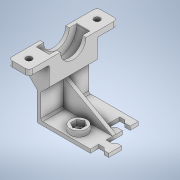
# Autodesk Inventor part: ДержательПодшипника_БН
Saved by Autodesk Inventor 2021 (Build 250183000, 183)
## iProperties
Created: 2023-02-11
Part Number: ДержательПодшипника_БН
Material: Типовые
Document SubType Name: Modeling
Designer: 1
Density: 1 g/cm^3
Appearance: По умолчанию
Author: 1
Autodesk Inventor part; units mm, degrees
ref_plane "YZ Plane" through (0, 0, 0) normal (1, 0, 0) x (0, 1, 0)
ref_plane "XZ Plane" through (0, 0, 0) normal (0, 1, 0) x (-1, 0, 0)
ref_plane "XY Plane" through (0, 0, 0) normal (0, 0, 1) x (1, 0, 0)
sketch "Эскиз1" plane through (0, 0, 0) normal (0, 0, 1) x (1, 0, 0)
  line L0 (0, 0) -> (-2, 0)
  line L1 (-2, 0) -> (-2, 20)
  line L2 (-2, 20) -> (0, 20)
  line L3 (0, 20) -> (0, 0)
  line L4 (-2, 0) -> (27, 0)
  line L5 (27, 0) -> (27, 2)
  line L6 (27, 2) -> (-2, 2)
  line L7 (-2, 2) -> (-2, 0)
  point P0 (0, 2)
  dimension "d4" = 2
  dimension "d5" = 20
  dimension "d6" = 2
  dimension "d7" = 27
  constraints: 16 end point, 4 parallel, 2 horizontal, 2 perpendicular
  measures "d4" distance of L1.end L2.end
  measures "d5" distance of L0.end L1.end
  measures "d6" distance of L5.end L4.end
  measures "d7" distance between parallel lines of L5 L3
extrude "Выдавливание1" add sketch "Эскиз1" along normal mid plane 26.1
sketch "Эскиз2" plane through (-2, 20, 13.05) normal (0, 1, 0) x (1, 0, 0)
  line L0 (4.55, 2) -> (-2.55, 2) construction
  line L1 (-2.55, 2) -> (-2.55, 24.1) construction
  line L2 (-2.55, 24.1) -> (4.55, 24.1) construction
  line L3 (4.55, 24.1) -> (4.55, 2) construction
  line L4 (4.55, 2) -> (-2.55, 24.1) construction
  line L5 (-2.55, 2) -> (4.55, 24.1) construction
  line L6 (2, 26.1) -> (2, 0) construction
  line L7 (0, 0) -> (0, 26.1) construction
  line L8 (2, 0) -> (0, 0) construction
  line L9 (2, 26.1) -> (2, 0) construction
  line L10 (0, 26.1) -> (2, 26.1) construction
  line L11 (6.55, 26.1) -> (-4.55, 26.1)
  line L12 (-4.55, 26.1) -> (-4.55, 0)
  line L13 (-4.55, 0) -> (6.55, 0)
  line L14 (6.55, 0) -> (6.55, 26.1)
  line L15 (6.55, 26.1) -> (-4.55, 0) construction
  line L16 (-4.55, 26.1) -> (6.55, 0) construction
  point P0 (2, 13.05)
  point P1 (1, 13.05)
  point P2 (1, 13.05)
  point P3 (2, 13.05)
  point P4 (1, 13.05)
  point P5 (1, 26.1)
  dimension "d10" = 7.1
  dimension "d11" = 22.1
  dimension "d12" = 2
  dimension "d13" = 2
  constraints: 24 end point, 8 midpoint, 4 parallel, 2 horizontal, 2 perpendicular, 1 horizontal alignment, 1 vertical alignment
  measures "d10" distance of L0.start L0.end
  measures "d11" distance of L0.end L1.end
  measures "d12" distance between parallel lines of L11 L2
  measures "d13" distance between parallel lines of L3 L14
extrude "Выдавливание2" add sketch "Эскиз2" along normal blind 13.5
shell "Оболочка1" thickness 2 removed faces 1 at (0.85, 33.5, -4.35)
fillet "Сопряжение1" radius 11 6 edges at (1.275, 22, -11.05) (-1, 22, -11.05) (-3.275, 22, -11.05) (-3.275, 22, 11.05) (-1, 22, 11.05) (1.275, 22, 11.05)
sketch "Эскиз3" plane through (-6.55, 20, -13.05) normal (-1, 0, 0) x (0, 0, 1)
  line L0 (26.1, 13.5) -> (0, 13.5) projected
  circle A0 centre (13.05, 13.5) radius 7
  point P0 (13.05, -20)
  point P1 (6.05, 13.5)
  point P2 (20.05, 13.5)
  dimension "d18" = 14
  constraints: 1 centre point, 1 midpoint
  measures "d18" diameter of A0
extrude "Выдавливание3" cut sketch "Эскиз3" against normal through all contours A0 L0 picked at (11.6567, 11.0213)
sketch "Эскиз4" plane through (0, 2, 13.05) normal (0, 1, 0) x (1, 0, 0)
  line L0 (27, 26.1) -> (27, 0) projected
  line L1 (27, 17.575) -> (24, 17.575)
  line L2 (24, 17.575) -> (22.5, 16.075)
  line L3 (22.5, 16.075) -> (20, 16.075)
  line L4 (27, 19.575) -> (10.0579, 19.575)
  line L5 (20, 16.075) -> (20, 19.575)
  line L6 (27, 21.575) -> (24, 21.575)
  line L7 (24, 21.575) -> (22.5, 23.075)
  line L8 (22.5, 23.075) -> (20, 23.075)
  line L9 (20, 23.075) -> (20, 19.575)
  line L10 (27, 13.05) -> (4.55, 13.05)
  line L11 (0, 26.1) -> (27, 26.1) projected
  line L12 (9.0322, 13.05) -> (9.0322, 26.1) construction
  line L13 (4.55, 20.05) -> (4.55, 6.05) projected
  line L14 (27, 8.525) -> (24, 8.525) construction
  line L15 (24, 8.525) -> (22.5, 10.025) construction
  line L16 (22.5, 10.025) -> (20, 10.025) construction
  line L17 (27, 6.525) -> (10.0579, 6.525)
  line L18 (20, 10.025) -> (20, 6.525) construction
  line L19 (27, 4.525) -> (24, 4.525) construction
  line L20 (24, 4.525) -> (22.5, 3.025) construction
  line L21 (22.5, 3.025) -> (20, 3.025) construction
  line L22 (20, 3.025) -> (20, 6.525) construction
  line L23 (31.5, 10.025) -> (34, 10.025)
  line L24 (30, 8.525) -> (31.5, 10.025)
  line L25 (27, 8.525) -> (30, 8.525)
  line L26 (34, 10.025) -> (34, 6.525)
  line L27 (27, 6.525) -> (43.9421, 6.525)
  line L28 (27, 4.525) -> (30, 4.525)
  line L29 (34, 3.025) -> (34, 6.525)
  line L30 (31.5, 3.025) -> (34, 3.025)
  line L31 (30, 4.525) -> (31.5, 3.025)
  line L32 (27, 4.525) -> (27, 8.525)
  line L33 (27, 17.575) -> (27, 21.575)
  point P0 (0, 13.05)
  point P1 (9.0322, 19.575)
  dimension "d21" = 3
  dimension "d22" = 7
  dimension "d23" = 2.5
  dimension "d24" = 4
  dimension "d25" = 7
  constraints: 62 end point, 23 symmetric about line, 7 point on line, 3 midpoint, 2 collinear, 2 horizontal, 2 perpendicular, 1 horizontal alignment, 1 parallel
  measures "d21" distance of L1.start L1.end
  measures "d22" distance between parallel lines of L8 L3
  measures "d23" distance of L2.end L3.end
  measures "d24" distance between parallel lines of L6 L1
  measures "d25" distance between parallel lines of L0 L9
extrude "Выдавливание4" add sketch "Эскиз4" against normal up to surface (2 mm away) contours L25 L24 L23 L26 L27 L0 | L27 L29 L30 L31 L28 L0
extrude "Выдавливание5" cut sketch "Эскиз4" against normal through all contours L0 L4 L9 L8 L7 L6 | L0 L1 L2 L3 L5 L4
sketch "Эскиз5" plane through (0, 0, 0) normal (0, 0, 1) x (1, 0, 0)
  line L0 (0, 17) -> (27, 2)
  point P0 (0, 0)
  point P1 (0, 20)
  dimension "d65" = 15
  constraints: 2 end point, 1 coincident, 1 vertical alignment
  measures "d65" vertical distance of L0.start L0.end
extrude "Ребро жесткости1" add sketch "Эскиз5" along normal mid plane 2 rib yes fills toward (13.4757, 9.4563) open curves L0
sketch "Эскиз6" plane through (-2, 33.5, 13.05) normal (0, 1, 0) x (1, 0, 0)
  line L0 (-4.55, 6.05) -> (-4.55, 20.05) projected
  line L1 (-4.55, 13.05) -> (30.5644, 13.05)
  line L2 (-4.55, 6.05) -> (-4.55, 0) projected
  line L3 (-4.55, 0) -> (6.55, 0)
  line L4 (6.55, 0) -> (6.55, -11.1)
  line L5 (6.55, -11.1) -> (-4.55, -11.1)
  line L6 (-4.55, -11.1) -> (-4.55, 0)
  circle A0 centre (1, -5.55) radius 1.6
  line L7 (-4.55, 26.1) -> (6.55, 26.1)
  line L8 (6.55, 26.1) -> (6.55, 37.2)
  line L9 (6.55, 37.2) -> (-4.55, 37.2)
  line L10 (-4.55, 37.2) -> (-4.55, 26.1)
  circle A1 centre (1, 31.65) radius 1.6
  point P0 (2, 13.05)
  point P1 (1, -11.1)
  point P2 (6.55, -5.55)
  point P3 (1, 37.2)
  point P4 (6.55, 31.65)
  dimension "d36" = 3.2
  constraints: 18 end point, 8 symmetric about line, 3 midpoint, 2 centre point, 2 coincident, 2 horizontal, 2 parallel, 2 perpendicular, 1 horizontal alignment, 1 vertical alignment, 1 other
  measures "d36" diameter of A0
extrude "Выдавливание6" add sketch "Эскиз6" against normal blind 3
fillet "Сопряжение2" radius 1 4 edges at (-1, 30.5, 13.05) (-1, 30.5, -13.05) (0, 2, -7.025) (0, 2, 7.025)
fillet "Сопряжение3" radius 0.5 1 edges at (-2, 0, 0)
chamfer "Фаска1" distance 4.55 angle 45 2 edges at (0, 20, 0) (-2, 20, 0)
sketch "Эскиз7" plane through (24, 2, -4.525) normal (0, 1, 0) x (1, 0, 0)
  line L0 (-4, -1.5) -> (-4, 5.5) projected
  line L1 (-1.5, -1.5) -> (-4, -1.5) projected
  line L2 (0, 0) -> (-1.5, -1.5) projected
  line L3 (3, 0) -> (0, 0) projected
  line L4 (0, 4) -> (3, 4) projected
  line L5 (-1.5, 5.5) -> (0, 4) projected
  line L6 (-4, 5.5) -> (-1.5, 5.5) projected
  line L7 (3, 0) -> (3, -3.525) projected
  line L8 (3, -0.1) -> (0.0414, -0.1)
  line L9 (0.0414, -0.1) -> (-1.4586, -1.6)
  line L10 (-1.4586, -1.6) -> (-4.1, -1.6)
  line L11 (-4.1, -1.6) -> (-4.1, 5.6)
  line L12 (-4.1, 5.6) -> (-1.4586, 5.6)
  line L13 (-1.4586, 5.6) -> (0.0414, 4.1)
  line L14 (0.0414, 4.1) -> (3, 4.1)
  line L15 (3, 8.525) -> (3, 4) projected
  point P0 (-24, -4.525)
  dimension "d44" = 0.1
  dimension "d45" = 0.1
  dimension "d46" = 0.1
  dimension "d47" = 0.1
  dimension "d48" = 0.1
  dimension "d49" = 0.1
  dimension "d50" = 0.1
  constraints: 14 end point, 4 parallel, 3 perpendicular, 2 point on line, 1 horizontal
  measures "d44" distance between parallel lines of L3 L8
  measures "d45" distance between parallel lines of L2 L9
  measures "d46" distance between parallel lines of L1 L10
  measures "d47" distance between parallel lines of L11 L0
  measures "d48" distance between parallel lines of L12 L6
  measures "d49" distance between parallel lines of L13 L5
  measures "d50" distance between parallel lines of L4 L14
extrude "Выдавливание7" cut sketch "Эскиз7" against normal through all
sketch "Эскиз8" plane through (1, 2, -13.05) normal (0, 1, 0) x (1, 0, 0)
  line L0 (26, -12.05) -> (26, -14.05) projected
  circle A0 centre (14, -20.55) radius 4.5
  line L1 (26, -21.575) -> (26, -26.1) projected
  line L2 (-1, -14.05) -> (-1, -26.1) projected
  line L3 (11.15, -18.9046) -> (14, -17.2591)
  line L4 (14, -17.2591) -> (16.85, -18.9046)
  line L5 (16.85, -18.9046) -> (16.85, -22.1954)
  line L6 (16.85, -22.1954) -> (14, -23.8409)
  line L7 (14, -23.8409) -> (11.15, -22.1954)
  line L8 (11.15, -22.1954) -> (11.15, -18.9046)
  line L9 (-7.55, 0) -> (-7.55, -26.1) projected
  point P0 (-1, -13.05)
  point P1 (-7.55, -13.05)
  dimension "d53" = 9
  dimension "d55" = 15
  dimension "d57" = 5.7
  dimension "d58" = 7.5
  constraints: 12 end point, 1 centre point, 1 coincident, 1 midpoint, 1 vertical, 13 other
  measures "d53" diameter of A0
  measures "d55" distance from line of L2 A0.centre
  measures "d57" distance between parallel lines of L8 L5
  measures "d58" vertical distance of A0.centre point (-7.55, -13.05)
extrude "Выдавливание8" add sketch "Эскиз8" along normal blind 3
sketch "Эскиз9" plane through (12.15, 2, 9.1454) normal (0, 1, 0) x (1, 0, 0)
  circle A0 centre (2.85, 1.6454) radius 1.6
  circle A1 centre (2.85, 1.6454) radius 4.5 projected
  point P0 (-12.15, 9.1454)
  dimension "d61" = 3.2
  constraints: 1 centre point, 1 concentric
  measures "d61" diameter of A0
extrude "Выдавливание9" cut sketch "Эскиз9" against normal through all contours A0
fillet "Сопряжение4" radius 2 4 edges at (4.55, 32, 24.15) (-6.55, 32, 24.15) (-6.55, 32, -24.15) (4.55, 32, -24.15)
